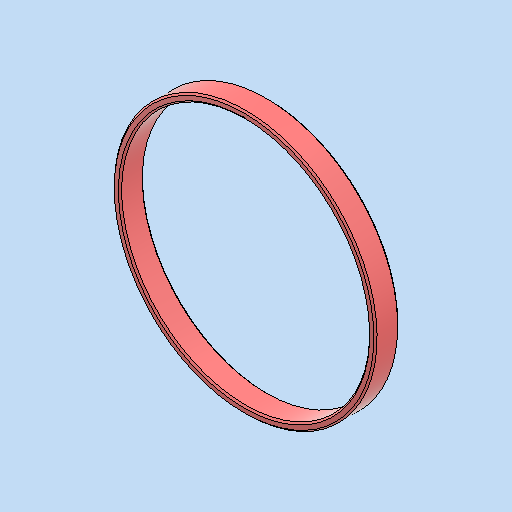
# Autodesk Inventor part: light-seam
Saved by Autodesk Inventor 2025 (Build 290162000, 162)
## iProperties
Created: 2025-02-18
Part Number: light-seam
Material: ABS Plastic
Document SubType Name: Modeling
Designer: kuzmin
Density: 1.06 g/cm^3
Appearance: Smooth - Red
Author: kuzmin
Autodesk Inventor part; units mm, degrees
ref_plane "YZ Plane" through (0, 0, 0) normal (1, 0, 0) x (0, 1, 0)
ref_plane "XZ Plane" through (0, 0, 0) normal (0, 1, 0) x (-1, 0, 0)
ref_plane "XY Plane" through (0, 0, 0) normal (0, 0, 1) x (1, 0, 0)
sketch "Sketch1" plane through (0, 0, 0) normal (0, 0, 1) x (1, 0, 0)
  circle A0 centre (0, 0) radius 30.1
  circle A1 centre (0, 0) radius 31.9
  dimension "d0" = 60.2
  dimension "d1" = 63.8
  constraints: 2 centre point, 2 coincident
  measures "d0" diameter of A0
  measures "d1" diameter of A1
extrude "Extrusion1" add sketch "Sketch1" along normal blind 5.8
sketch "Sketch2" plane through (0, 0, 5.8) normal (0, 0, 1) x (1, 0, 0)
  line L0 (-0.15, 30.6) -> (0.15, 30.6)
  line L1 (0.15, 30.6) -> (0.15, 28.6)
  line L2 (0.15, 28.6) -> (-0.15, 28.6)
  line L3 (-0.15, 28.6) -> (-0.15, 30.6)
  line L4 (-0.15, -33.5) -> (0.15, -33.5)
  line L5 (0.15, -33.5) -> (0.15, -31.5)
  line L6 (0.15, -31.5) -> (-0.15, -31.5)
  line L7 (-0.15, -31.5) -> (-0.15, -33.5)
  point P0 (0, 0)
  point P1 (0, 28.6)
  point P2 (0, -31.5)
  dimension "d7" = 30.6
  dimension "d8" = 0.3
  dimension "d9" = 2
  dimension "d10" = 31.5
  dimension "d11" = 2
  constraints: 16 end point, 4 parallel, 2 horizontal, 2 midpoint, 2 perpendicular, 2 vertical alignment, 1 point on line
  measures "d7" distance from line of point (0, 0) L0
  measures "d8" distance of L1.end L2.end
  measures "d9" distance of L2.end L0.start
  measures "d10" distance of point (0, 0) point (0, -31.5)
  measures "d11" distance of L4.end L5.end
extrude "Extrusion2" cut sketch "Sketch2" against normal through all
chamfer "Chamfer1" distance 0.4 angle 45 8 edges at (-22.5036, 22.6097, 5.8) (22.6097, -22.5036, 5.8) (21.3369, 21.2308, 5.8) (-21.2308, -21.3369, 5.8) (-22.5036, 22.6097, 0) (22.6097, -22.5036, 0) (21.3369, 21.2308, 0) (-21.2308, -21.3369, 0)
body "Solid1"
